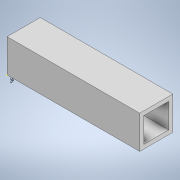
# Autodesk Inventor part: Side Piece
Saved by Autodesk Inventor 2022 (Build 260153000, 153)
## iProperties
Created: 2022-01-02
Part Number: Side Piece
Material: Generic
Document SubType Name: Modeling
Designer: josephinew
Density: 1 g/cm^3
Appearance: Default
Author: josephinew
Autodesk Inventor part; units mm, degrees
ref_plane "YZ Plane" through (0, 0, 0) normal (1, 0, 0) x (0, 1, 0)
ref_plane "XZ Plane" through (0, 0, 0) normal (0, 1, 0) x (-1, 0, 0)
ref_plane "XY Plane" through (0, 0, 0) normal (0, 0, 1) x (1, 0, 0)
sketch "Sketch1" plane through (0, 0, 0) normal (1, 0, 0) x (0, 1, 0)
  point P0 (0, 0)
sketch "Sketch2" plane through (0, 0, 0) normal (1, 0, 0) x (0, 1, 0)
  line L0 (0, 0) -> (25.4, 0)
  line L1 (25.4, 0) -> (25.4, -25.4)
  line L2 (25.4, -25.4) -> (0, -25.4)
  line L3 (0, -25.4) -> (0, 0)
  dimension "d0" = 25.4
  dimension "d1" = 25.4
  constraints: 8 end point, 2 parallel, 1 horizontal, 1 perpendicular
  measures "d0" distance of L1.end L2.end
  measures "d1" distance of L0.end L1.end
extrude "Extrusion1" add sketch "Sketch2" along normal blind 101.6
sketch "Sketch3" plane through (101.6, 0, 0) normal (1, 0, 0) x (0, 0, -1)
  line L0 (0, 0) -> (25.4, 0) projected
  line L1 (0, 0) -> (3.175, 0)
  line L2 (3.175, 0) -> (0, 0)
  line L3 (3.175, 0) -> (3.175, 3.175)
  line L4 (3.175, 3.175) -> (22.225, 3.175)
  line L5 (22.225, 3.175) -> (22.225, 22.225)
  line L6 (22.225, 22.225) -> (3.175, 22.225)
  line L7 (3.175, 22.225) -> (3.175, 3.175)
  dimension "d7" = 19.05
  dimension "d8" = 19.05
  constraints: 14 end point, 2 parallel, 2 perpendicular, 1 collinear, 1 horizontal, 1 point on line
  measures "d7" distance of L6.end L5.end
  measures "d8" distance of L5.end L4.end
extrude "Extrusion2" cut sketch "Sketch3" against normal blind 50.8
sketch "Sketch4" plane through (0, 0, 0) normal (-1, 0, 0) x (0, 0, 1)
  line L0 (-25.4, 0) -> (-25.4, 25.4) projected
  line L1 (-25.4, 25.4) -> (0, 25.4) projected
  line L2 (-22.225, 3.175) -> (-3.175, 3.175) projected
  line L3 (-22.225, 22.225) -> (-22.225, 3.175) projected
  line L4 (-21.59, 3.302) -> (-22.098, 3.302)
  line L5 (-17.272, 8.128) -> (-8.128, 8.128)
  line L6 (-8.128, 8.128) -> (-8.128, 17.907)
  line L7 (-8.128, 17.907) -> (-17.272, 17.907)
  line L8 (-17.272, 17.907) -> (-17.272, 8.128)
  line L9 (-22.098, 3.302) -> (-3.302, 3.302)
  line L10 (-3.302, 3.302) -> (-3.302, 22.733)
  line L11 (-3.302, 22.733) -> (-22.098, 22.733)
  line L12 (-22.098, 22.733) -> (-22.098, 3.302)
  constraints: 18 end point, 4 parallel, 2 horizontal, 2 perpendicular
extrude "Extrusion3" cut sketch "Sketch4" against normal blind 38.1
body "Solid1"
